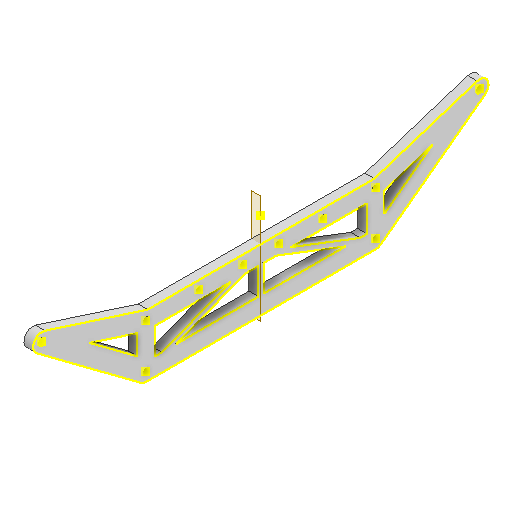
# Autodesk Inventor part: Horizontal_bar_V2
Saved by Autodesk Inventor 2022 (Build 260153000, 153)
## iProperties
Created: 2022-08-23
Part Number: Horizontal_bar_V2
Material: Generic
Document SubType Name: Modeling
Designer: dell
Density: 1 g/cm^3
Appearance: Default
Mass: 21.5376 g
Surface Area: 148.526 cm^2
Volume: 21.5376 cm^3
Author: dell
Autodesk Inventor part; units mm, degrees
ref_plane "YZ Plane" through (0, 0, 0) normal (1, 0, 0) x (0, 1, 0)
ref_plane "XZ Plane" through (0, 0, 0) normal (0, 1, 0) x (-1, 0, 0)
sketch "Sketch1" plane through (0, 0, 0) normal (1, 0, 0) x (0, 1, 0)
  circle A0 centre (0, -124) radius 1.95
  circle A1 centre (0, 124) radius 1.95
  circle A2 centre (-19, -65) radius 1.5
  circle A3 centre (-19, 65) radius 1.5
  line L0 (0, 124) -> (-19, 65) construction
  line L1 (4.7593, 122.4673) -> (-14.2407, 63.4673)
  line L2 (-23.7593, 66.5327) -> (-4.7593, 125.5327)
  arc A4 (4.7593, 122.4673) -> (-4.7593, 125.5327) centre (0, 124) ccw
  arc A5 (-23.7593, 66.5327) -> (-14.2407, 63.4673) centre (-19, 65) ccw
  line L3 (-19, 65) -> (-19, -65) construction
  line L4 (-24, 65) -> (-24, -65)
  line L5 (-14, -65) -> (-14, 65)
  arc A6 (-14, 65) -> (-24, 65) centre (-19, 65) ccw
  arc A7 (-24, -65) -> (-14, -65) centre (-19, -65) ccw
  line L6 (-19, -65) -> (0, -124) construction
  line L7 (-23.7593, -66.5327) -> (-4.7593, -125.5327)
  line L8 (4.7593, -122.4673) -> (-14.2407, -63.4673)
  arc A8 (-14.2407, -63.4673) -> (-23.7593, -66.5327) centre (-19, -65) ccw
  arc A9 (-4.7593, -125.5327) -> (4.7593, -122.4673) centre (0, -124) ccw
  circle A10 centre (-44, 65) radius 1.5
  circle A11 centre (-44, -65) radius 1.5
  line L9 (-19, 65) -> (-44, 65) construction
  line L10 (-19, 70) -> (-44, 70)
  line L11 (-44, 60) -> (-19, 60)
  arc A12 (-19, 60) -> (-19, 70) centre (-19, 65) ccw
  arc A13 (-44, 70) -> (-44, 60) centre (-44, 65) ccw
  line L12 (-19, -65) -> (-44, -65) construction
  line L13 (-19, -60) -> (-44, -60)
  line L14 (-44, -70) -> (-19, -70)
  arc A14 (-19, -70) -> (-19, -60) centre (-19, -65) ccw
  arc A15 (-44, -60) -> (-44, -70) centre (-44, -65) ccw
  line L15 (0, 124) -> (-44, 65) construction
  line L16 (-4.0081, 126.9891) -> (-48.0081, 67.9891)
  line L17 (-39.9919, 62.0109) -> (4.0081, 121.0109)
  arc A16 (4.0081, 121.0109) -> (-4.0081, 126.9891) centre (0, 124) ccw
  arc A17 (-48.0081, 67.9891) -> (-39.9919, 62.0109) centre (-44, 65) ccw
  line L18 (-44, -65) -> (0, -124) construction
  line L19 (-48.0081, -67.9891) -> (-4.0081, -126.9891)
  line L20 (4.0081, -121.0109) -> (-39.9919, -62.0109)
  arc A18 (-39.9919, -62.0109) -> (-48.0081, -67.9891) centre (-44, -65) ccw
  arc A19 (-4.0081, -126.9891) -> (4.0081, -121.0109) centre (0, -124) ccw
  line L21 (-44, 65) -> (-44, -65) construction
  line L22 (-49, 65) -> (-49, -65)
  line L23 (-39, -65) -> (-39, 65)
  arc A20 (-39, 65) -> (-49, 65) centre (-44, 65) ccw
  arc A21 (-49, -65) -> (-39, -65) centre (-44, -65) ccw
  line L24 (-44, 65) -> (-19, 0) construction
  line L25 (-45.4, 64.4615) -> (-20.4, -0.5385)
  line L26 (-17.6, 0.5385) -> (-42.6, 65.5385)
  arc A22 (-42.6, 65.5385) -> (-45.4, 64.4615) centre (-44, 65) ccw
  arc A23 (-20.4, -0.5385) -> (-17.6, 0.5385) centre (-19, 0) ccw
  line L27 (-44, -65) -> (-19, 0) construction
  line L28 (-42.6, -65.5385) -> (-17.6, -0.5385)
  line L29 (-20.4, 0.5385) -> (-45.4, -64.4615)
  arc A24 (-45.4, -64.4615) -> (-42.6, -65.5385) centre (-44, -65) ccw
  arc A25 (-17.6, -0.5385) -> (-20.4, 0.5385) centre (-19, 0) ccw
  line L30 (-19, 0) -> (-44, 0) construction
  line L31 (-19, 1.5) -> (-44, 1.5)
  line L32 (-44, -1.5) -> (-19, -1.5)
  arc A26 (-19, -1.5) -> (-19, 1.5) centre (-19, 0) ccw
  arc A27 (-44, 1.5) -> (-44, -1.5) centre (-44, 0) ccw
  circle A28 centre (-19, -10) radius 1.5
  circle A29 centre (-19, -35) radius 1.5
  circle A30 centre (-19, 10) radius 1.5
  circle A31 centre (-19, 35) radius 1.5
  point P0 (0, 0)
  point P1 (-9.5, 94.5)
  point P2 (-9.5, -94.5)
  point P3 (-14, -64.2148)
  point P4 (-14, 64.2148)
  point P5 (-24, 65)
  point P6 (-31.5, 65)
  point P7 (-31.5, -65)
  point P8 (-22, 94.5)
  point P9 (-22, -94.5)
  point P10 (-44, 0)
  point P11 (-31.5, 32.5)
  point P12 (-31.5, -32.5)
  point P13 (-39, 47.8215)
  point P14 (-24, 8.8215)
  point P15 (-24, 17.1785)
  point P16 (-40.4698, 60)
  point P17 (-24, 60)
  point P18 (-22.6427, 70)
  point P19 (-34.0339, 70)
  point P20 (-13.9854, 96.8832)
  point P21 (-6.8749, 118.9633)
  point P22 (-43.3898, 70)
  point P23 (-49, 65)
  point P24 (-43.3898, -70)
  point P25 (-6.8749, -118.9633)
  point P26 (-13.9854, -96.8832)
  point P27 (-34.0339, -70)
  point P28 (-22.6427, -70)
  point P29 (-24, -60)
  point P30 (-40.4698, -60)
  point P31 (-24, -17.1785)
  point P32 (-24, -8.8215)
  point P33 (-39, -47.8215)
  point P34 (-31.5, 0)
  point P35 (-39, -1.5)
  point P36 (-24, -1.5)
  point P37 (-24, 1.5)
  point P38 (-39, 1.5)
  point P39 (-49, 65)
  point P40 (-4.0081, -126.9891)
  point P41 (-39, 60)
  point P42 (-39, -60)
  point P43 (-39, -56.1785)
  point P44 (-39, 56.1785)
  dimension "d2" = 3.9
  dimension "d4" = 3.9
  dimension "d25" = 3
  dimension "d28" = 3
  dimension "d43" = 59
  dimension "d44" = 65
  dimension "d45" = 65
  dimension "d47" = 59
  dimension "d48" = 10
  dimension "d49" = 10
  dimension "d50" = 10
  dimension "d52" = 14
  dimension "d53" = 3
  dimension "d54" = 3
  dimension "d55" = 10
  dimension "d56" = 10
  dimension "d57" = 25
  dimension "d58" = 25
  dimension "d59" = 10
  dimension "d60" = 10
  dimension "d61" = 10
  dimension "d62" = 3
  dimension "d63" = 3
  dimension "d64" = 3
  dimension "d65" = 3
  dimension "d66" = 3
  dimension "d67" = 10
  dimension "d68" = 25
  dimension "d69" = 3
  dimension "d70" = 3
  dimension "d71" = 10
  dimension "d72" = 25
  constraints: 88 end point, 44 point on circle, 44 tangent, 32 centre point, 11 midpoint, 11 parallel, 4 point on line, 3 vertical alignment, 2 horizontal alignment, 1 coincident, 1 concentric, 1 horizontal, 1 perpendicular, 1 vertical
  measures "d2" diameter of A0
  measures "d4" diameter of A1
  measures "d25" diameter of A2
  measures "d28" diameter of A3
  measures "d43" vertical distance of L0.start L0.end
  measures "d44" vertical distance of point (0, 0) L0.end
  measures "d45" vertical distance of point (0, 0) L3.end
  measures "d47" vertical distance of L3.end L6.end
  measures "d48" distance between parallel lines of L1 L2
  measures "d49" distance between parallel lines of L4 L5
  measures "d50" distance between parallel lines of L7 L8
  measures "d52" distance from line of point (0, 0) L5
  measures "d53" diameter of A10
  measures "d54" diameter of A11
  measures "d55" diameter of A13
  measures "d56" diameter of A15
  measures "d57" distance of L0.end L9.end
  measures "d58" distance of L3.end L12.end
  measures "d59" diameter of A17
  measures "d60" diameter of A19
  measures "d61" diameter of A21
  measures "d62" diameter of A23
  measures "d63" diameter of A25
  measures "d64" diameter of A27
  measures "d65" diameter of A28
  measures "d66" diameter of A29
  measures "d67" distance of L24.end A28.centre
  measures "d68" distance of A28.centre A29.centre
  measures "d69" diameter of A30
  measures "d70" diameter of A31
  measures "d71" distance of L24.end A30.centre
  measures "d72" distance of A30.centre A31.centre
extrude "Extrusion1" add sketch "Sketch1" along normal blind 5 contours A16 L17 L2 A4 | L1 L5 A6 L10 L2 L17 A16 | L5 L8 A8 L13 L4 L28 A23 L26 L11 A5 L1 | L1 A12 L5 | A4 L2 L17 L10 A13 L16 | A5 A6 A12 | L8 A19 L20 L7 L14 A7 L5 | L5 A14 L8 | A13 A20 L23 L17 A17 L26 A10 L25 | L11 L4 A5 | A7 A8 A14 | A9 L7 L20 A19 | A6 L2 L10 | L10 L17 L23 A20 | A13 L11 L25 L23 L31 A27 L32 L29 L13 A15 L22 | L2 A5 L4 L11 L23 L17 L10 | L14 L7 A7 | L19 A15 L14 L20 L7 A9 | A8 L4 L13 | A17 L25 L11 | A15 A18 L29 A11 L28 L20 L23 A21 | L23 L11 L26 A17 L17 | L26 A25 L31 L25 L4 | L4 L25 L23 L26 | L23 L26 L11 | L7 L14 L20 L23 L13 L4 A7 | L25 A17 L26 L11 | L11 L26 L23 L25 | L25 A10 L26 A17 | L13 L29 A18 | L25 L31 L4 | A23 L25 L29 A25 | L14 A21 L23 L20 | L28 L23 L29 L4 | L4 L29 L32 A23 L28 | L23 L20 A18 L28 L13 | L13 L28 L23 | L29 L23 L28 L13 | L13 L28 A18 L29 | A18 L28 A11 L29 | L31 L25 L29 L32 L4 | L4 L32 L23 L31 | L31 A25 L29 L25 | L4 L32 L29 | L23 L32 A27 L31 | L25 A23 L32 L29
sketch "Sketch7" plane through (5, 0, 0) normal (1, 0, 0) x (0, 0, -1)
  circle A0 centre (-65, -19) radius 1.5 projected
  circle A1 centre (-35, -19) radius 1.5 projected
  circle A2 centre (-10, -19) radius 1.5 projected
  circle A3 centre (35, -19) radius 1.5 projected
  circle A4 centre (10, -19) radius 1.5 projected
  circle A5 centre (65, -19) radius 1.5 projected
  circle A6 centre (124, 0) radius 1.95 projected
  line L0 (-17.1785, -24) -> (-56.1785, -39) projected
  line L1 (-56.1785, -39) -> (-60, -39) projected
  line L2 (-60, -39) -> (-60, -24) projected
  line L3 (-60, -24) -> (-17.1785, -24) projected
  circle A7 centre (65, -44) radius 1.5 projected
  circle A8 centre (-65, -44) radius 1.5 projected
  line L4 (-96.8832, -13.9854) -> (-70, -22.6427) projected
  line L5 (-70, -22.6427) -> (-70, -34.0339) projected
  line L6 (-70, -34.0339) -> (-96.8832, -13.9854) projected
  line L7 (-1.5, -39) -> (-47.8215, -39) projected
  line L8 (-47.8215, -39) -> (-8.8215, -24) projected
  line L9 (-8.8215, -24) -> (-1.5, -24) projected
  line L10 (-1.5, -24) -> (-1.5, -39) projected
  line L11 (8.8215, -24) -> (47.8215, -39) projected
  line L12 (47.8215, -39) -> (1.5, -39) projected
  line L13 (1.5, -39) -> (1.5, -24) projected
  line L14 (1.5, -24) -> (8.8215, -24) projected
  line L15 (60, -24) -> (60, -39) projected
  line L16 (60, -39) -> (56.1785, -39) projected
  line L17 (56.1785, -39) -> (17.1785, -24) projected
  line L18 (17.1785, -24) -> (60, -24) projected
  line L19 (96.8832, -13.9854) -> (70, -34.0339) projected
  line L20 (70, -34.0339) -> (70, -22.6427) projected
  line L21 (70, -22.6427) -> (96.8832, -13.9854) projected
  arc A9 (126.9891, -4.0081) -> (122.4673, 4.7593) centre (124, 0) ccw projected
  line L22 (122.4673, 4.7593) -> (64.2148, -14) projected
  line L23 (64.2148, -14) -> (-64.2148, -14) projected
  line L24 (-64.2148, -14) -> (-122.4673, 4.7593) projected
  arc A10 (-122.4673, 4.7593) -> (-126.9891, -4.0081) centre (-124, 0) ccw projected
  line L25 (-126.9891, -4.0081) -> (-67.9891, -48.0081) projected
  arc A11 (-67.9891, -48.0081) -> (-65, -49) centre (-65, -44) ccw projected
  line L26 (-65, -49) -> (65, -49) projected
  arc A12 (65, -49) -> (67.9891, -48.0081) centre (65, -44) ccw projected
  line L27 (67.9891, -48.0081) -> (126.9891, -4.0081) projected
  circle A13 centre (-124, 0) radius 1.95 projected
  point P0 (0, 0)
body "Solid1"
